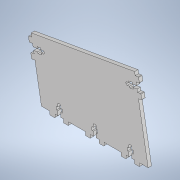
# Autodesk Inventor part: tc_support_down
Saved by Autodesk Inventor 2020 (Build 240168000, 168)
## iProperties
Created: 2019-07-16
Part Number: tc_support_down
Material: Générique
Document SubType Name: Modeling
Designer: Thibault
Density: 1 g/cm^3
Appearance: Par défaut
Author: Thibault
Autodesk Inventor part; units mm, degrees
ref_plane "YZ Plane" through (0, 0, 0) normal (1, 0, 0) x (0, 1, 0)
ref_plane "XZ Plane" through (0, 0, 0) normal (0, 1, 0) x (-1, 0, 0)
ref_plane "XY Plane" through (0, 0, 0) normal (0, 0, 1) x (1, 0, 0)
sketch "Anchor (screw side)" plane through (0, 0, 0) normal (0, 0, 1) x (1, 0, 0)
  circle A0 centre (93.7814, 50.2592) radius 0.85
  line L0 (91.2814, 51.2592) -> (88.2814, 51.2592)
  line L1 (88.2814, 51.2592) -> (88.2814, 49.2592)
  line L2 (88.2814, 49.2592) -> (91.2814, 49.2592)
  line L3 (91.2814, 49.2592) -> (91.2814, 51.2592)
  line L4 (99.2814, 51.2592) -> (96.2814, 51.2592)
  line L5 (96.2814, 51.2592) -> (96.2814, 49.2592)
  line L6 (96.2814, 49.2592) -> (99.2814, 49.2592)
  line L7 (99.2814, 49.2592) -> (99.2814, 51.2592)
  line L8 (91.2814, 51.2592) -> (96.2814, 49.2592) construction
  line L9 (96.2814, 51.2592) -> (91.2814, 49.2592) construction
  line L10 (86.6814, 52.8592) -> (100.8814, 52.8592) construction
  line L11 (100.8814, 52.8592) -> (100.8814, 47.6592) construction
  line L12 (100.8814, 47.6592) -> (86.6814, 47.6592) construction
  line L13 (86.6814, 47.6592) -> (86.6814, 52.8592) construction
  point P0 (103.5798, 50.1132)
  dimension "d27" = 1.7
  dimension "d28" = 3
  dimension "d29" = 2
  dimension "d30" = 3
  dimension "d32" = 5
  dimension "d34" = 1.6
  dimension "d35" = 1.6
  dimension "d36" = 1.6
  dimension "d37" = 1.6
  measures "d27" diameter of A0
  measures "d28" distance of L2.end L1.end
  measures "d29" distance of L1.end L0.end
  measures "d30" distance of L6.end L5.end
  measures "d32" distance between parallel lines of L5 L3
  measures "d34" distance between parallel lines of L0 L10
  measures "d35" distance between parallel lines of L12 L2
  measures "d36" distance between parallel lines of L11 L7
  measures "d37" distance between parallel lines of L13 L1
sketch "Anchor (nut side)" plane through (0, 0, 0) normal (0, 0, 1) x (1, 0, 0)
  line L0 (10, 0) -> (8.35, 0)
  line L1 (8.35, 0) -> (8.35, -2.5)
  line L2 (8.35, -2.5) -> (9.15, -2.5)
  line L3 (9.15, -2.5) -> (9.15, -4.5)
  line L4 (5.85, -4.5) -> (5.85, -2.5)
  line L5 (5.85, -2.5) -> (6.65, -2.5)
  line L6 (6.65, -2.5) -> (6.65, 0)
  line L7 (6.65, 0) -> (5, 0)
  line L8 (2, 0) -> (2, 1.75)
  line L9 (2, 0) -> (3, 0) construction
  line L10 (2.25, 2) -> (4.75, 2)
  line L11 (5, 1.75) -> (5, 0)
  line L12 (5, 2) -> (7, 2) construction
  line L13 (10, 0) -> (10, 1.75)
  line L14 (10.25, 2) -> (12.75, 2)
  line L15 (13, 1.75) -> (13, 0)
  line L16 (0, 0) -> (2, 0)
  line L17 (13, 0) -> (15, 0)
  line L18 (5.85, -4.5) -> (6.65, -4.5)
  line L19 (9.15, -4.5) -> (8.35, -4.5)
  line L20 (6.65, -4.5) -> (6.65, -6)
  line L21 (8.35, -4.5) -> (8.35, -6)
  arc A0 (2.25, 2) -> (2, 1.75) centre (2.25, 1.75) ccw
  arc A1 (5, 1.75) -> (4.75, 2) centre (4.75, 1.75) ccw
  arc A2 (10.25, 2) -> (10, 1.75) centre (10.25, 1.75) ccw
  arc A3 (13, 1.75) -> (12.75, 2) centre (12.75, 1.75) ccw
  line L22 (7.15, -6.5) -> (7.85, -6.5)
  arc A4 (6.65, -6) -> (7.15, -6.5) centre (7.15, -6) ccw
  arc A5 (7.85, -6.5) -> (8.35, -6) centre (7.85, -6) ccw
  point P0 (9.1321, -0.6227)
  point P1 (2, 2)
  point P2 (10, 2)
  point P3 (13, 2)
  point P4 (6.65, -6.5)
  point P5 (8.35, -6.5)
  dimension "d3" = 2
  dimension "d5" = 3
  dimension "d7" = 5
  dimension "d8" = 3
  dimension "d10" = 1.65
  dimension "d11" = 2.5
  dimension "d12" = 0.8
  dimension "d13" = 2
  dimension "d14" = 0.8
  dimension "d15" = 1.7
  dimension "d16" = 2.5
  dimension "d18" = 2
  dimension "d19" = 0.8
  dimension "d20" = 0.8
  dimension "d21" = 2
  dimension "d22" = 2
  dimension "d23" = 1.7
  dimension "d24" = 2
  dimension "d25" = 0.25
  dimension "d38" = 2
  dimension "d39" = 0.5
  measures "d3" distance of point (0, 0) L8.start
  measures "d5" distance of point (2, 2) L12.start
  measures "d7" distance of L7.end L0.start
  measures "d8" distance of point (10, 2) point (13, 2)
  measures "d10" distance of L0.start L0.end
  measures "d11" distance of L0.end L1.end
  measures "d12" distance of L1.end L2.end
  measures "d13" distance of L2.end L3.end
  measures "d14" distance of L4.end L5.end
  measures "d15" distance of L6.end L0.end
  measures "d16" distance of L5.end L6.end
  measures "d18" distance of L15.end point (15, 0)
  measures "d19" distance of L4.start L18.end
  measures "d20" distance of L3.end L19.end
  measures "d21" distance of L18.end point (6.65, -6.5)
  measures "d22" distance of L19.end point (8.35, -6.5)
  measures "d23" distance of L18.end L19.end
  measures "d24" distance of L4.start L4.end
  measures "d25" radius of A0
  measures "d38" distance of the line from the sketch origin of L10
  measures "d39" radius of A4
derived "shared_parameters.ipt"
sketch "Esquisse2" plane through (0, 0, 0) normal (0, 0, 1) x (1, 0, 0)
  line L0 (-14.577, 4.8239) -> (-8.577, 4.8239)
  line L1 (6.423, 4.8239) -> (12.423, 4.8239)
  line L2 (-29.577, 4.8239) -> (-32.577, 4.8239)
  line L3 (27.423, 4.8239) -> (30.423, 4.8239)
  line L4 (-32.577, 4.8239) -> (-32.577, 9.8239)
  line L5 (-32.577, 24.8239) -> (30.423, 24.8239)
  line L6 (30.423, 9.8239) -> (30.423, 4.8239)
  line L7 (-24.577, 4.8239) -> (-22.927, 4.8239)
  line L8 (-22.927, 4.8239) -> (-22.927, 7.3239)
  line L9 (-22.927, 7.3239) -> (-23.727, 7.3239)
  line L10 (-23.727, 7.3239) -> (-23.727, 9.3239)
  line L11 (-20.427, 9.3239) -> (-20.427, 7.3239)
  line L12 (-20.427, 7.3239) -> (-21.227, 7.3239)
  line L13 (-21.227, 7.3239) -> (-21.227, 4.8239)
  line L14 (-21.227, 4.8239) -> (-19.577, 4.8239)
  line L15 (-16.577, 4.8239) -> (-16.577, 3.0739)
  line L16 (-16.577, 4.8239) -> (-17.577, 4.8239) construction
  line L17 (-16.827, 2.8239) -> (-19.327, 2.8239)
  line L18 (-19.577, 3.0739) -> (-19.577, 4.8239)
  line L19 (-19.577, 2.8239) -> (-21.577, 2.8239) construction
  line L20 (-24.577, 4.8239) -> (-24.577, 3.0739)
  line L21 (-24.827, 2.8239) -> (-27.327, 2.8239)
  line L22 (-27.577, 3.0739) -> (-27.577, 4.8239)
  line L23 (-14.577, 4.8239) -> (-16.577, 4.8239)
  line L24 (-27.577, 4.8239) -> (-29.577, 4.8239)
  line L25 (-20.427, 9.3239) -> (-21.227, 9.3239)
  line L26 (-23.727, 9.3239) -> (-22.927, 9.3239)
  line L27 (-21.227, 9.3239) -> (-21.227, 10.8239)
  line L28 (-22.927, 9.3239) -> (-22.927, 10.8239)
  arc A0 (-16.827, 2.8239) -> (-16.577, 3.0739) centre (-16.827, 3.0739) ccw
  arc A1 (-19.577, 3.0739) -> (-19.327, 2.8239) centre (-19.327, 3.0739) ccw
  arc A2 (-24.827, 2.8239) -> (-24.577, 3.0739) centre (-24.827, 3.0739) ccw
  arc A3 (-27.577, 3.0739) -> (-27.327, 2.8239) centre (-27.327, 3.0739) ccw
  line L29 (-21.727, 11.3239) -> (-22.427, 11.3239)
  arc A4 (-21.227, 10.8239) -> (-21.727, 11.3239) centre (-21.727, 10.8239) ccw
  arc A5 (-22.427, 11.3239) -> (-22.927, 10.8239) centre (-22.427, 10.8239) ccw
  line L30 (-3.577, 4.8239) -> (-1.927, 4.8239)
  line L31 (-1.927, 4.8239) -> (-1.927, 7.3239)
  line L32 (-1.927, 7.3239) -> (-2.727, 7.3239)
  line L33 (-2.727, 7.3239) -> (-2.727, 9.3239)
  line L34 (0.573, 9.3239) -> (0.573, 7.3239)
  line L35 (0.573, 7.3239) -> (-0.227, 7.3239)
  line L36 (-0.227, 7.3239) -> (-0.227, 4.8239)
  line L37 (-0.227, 4.8239) -> (1.423, 4.8239)
  line L38 (4.423, 4.8239) -> (4.423, 3.0739)
  line L39 (4.423, 4.8239) -> (3.423, 4.8239) construction
  line L40 (4.173, 2.8239) -> (1.673, 2.8239)
  line L41 (1.423, 3.0739) -> (1.423, 4.8239)
  line L42 (1.423, 2.8239) -> (-0.577, 2.8239) construction
  line L43 (-3.577, 4.8239) -> (-3.577, 3.0739)
  line L44 (-3.827, 2.8239) -> (-6.327, 2.8239)
  line L45 (-6.577, 3.0739) -> (-6.577, 4.8239)
  line L46 (6.423, 4.8239) -> (4.423, 4.8239)
  line L47 (-6.577, 4.8239) -> (-8.577, 4.8239)
  line L48 (0.573, 9.3239) -> (-0.227, 9.3239)
  line L49 (-2.727, 9.3239) -> (-1.927, 9.3239)
  line L50 (-0.227, 9.3239) -> (-0.227, 10.8239)
  line L51 (-1.927, 9.3239) -> (-1.927, 10.8239)
  arc A6 (4.173, 2.8239) -> (4.423, 3.0739) centre (4.173, 3.0739) ccw
  arc A7 (1.423, 3.0739) -> (1.673, 2.8239) centre (1.673, 3.0739) ccw
  arc A8 (-3.827, 2.8239) -> (-3.577, 3.0739) centre (-3.827, 3.0739) ccw
  arc A9 (-6.577, 3.0739) -> (-6.327, 2.8239) centre (-6.327, 3.0739) ccw
  line L52 (-0.727, 11.3239) -> (-1.427, 11.3239)
  arc A10 (-0.227, 10.8239) -> (-0.727, 11.3239) centre (-0.727, 10.8239) ccw
  arc A11 (-1.427, 11.3239) -> (-1.927, 10.8239) centre (-1.427, 10.8239) ccw
  line L53 (17.423, 4.8239) -> (19.073, 4.8239)
  line L54 (19.073, 4.8239) -> (19.073, 7.3239)
  line L55 (19.073, 7.3239) -> (18.273, 7.3239)
  line L56 (18.273, 7.3239) -> (18.273, 9.3239)
  line L57 (21.573, 9.3239) -> (21.573, 7.3239)
  line L58 (21.573, 7.3239) -> (20.773, 7.3239)
  line L59 (20.773, 7.3239) -> (20.773, 4.8239)
  line L60 (20.773, 4.8239) -> (22.423, 4.8239)
  line L61 (25.423, 4.8239) -> (25.423, 3.0739)
  line L62 (25.423, 4.8239) -> (24.423, 4.8239) construction
  line L63 (25.173, 2.8239) -> (22.673, 2.8239)
  line L64 (22.423, 3.0739) -> (22.423, 4.8239)
  line L65 (22.423, 2.8239) -> (20.423, 2.8239) construction
  line L66 (17.423, 4.8239) -> (17.423, 3.0739)
  line L67 (17.173, 2.8239) -> (14.673, 2.8239)
  line L68 (14.423, 3.0739) -> (14.423, 4.8239)
  line L69 (27.423, 4.8239) -> (25.423, 4.8239)
  line L70 (14.423, 4.8239) -> (12.423, 4.8239)
  line L71 (21.573, 9.3239) -> (20.773, 9.3239)
  line L72 (18.273, 9.3239) -> (19.073, 9.3239)
  line L73 (20.773, 9.3239) -> (20.773, 10.8239)
  line L74 (19.073, 9.3239) -> (19.073, 10.8239)
  arc A12 (25.173, 2.8239) -> (25.423, 3.0739) centre (25.173, 3.0739) ccw
  arc A13 (22.423, 3.0739) -> (22.673, 2.8239) centre (22.673, 3.0739) ccw
  arc A14 (17.173, 2.8239) -> (17.423, 3.0739) centre (17.173, 3.0739) ccw
  arc A15 (14.423, 3.0739) -> (14.673, 2.8239) centre (14.673, 3.0739) ccw
  line L75 (20.273, 11.3239) -> (19.573, 11.3239)
  arc A16 (20.773, 10.8239) -> (20.273, 11.3239) centre (20.273, 10.8239) ccw
  arc A17 (19.573, 11.3239) -> (19.073, 10.8239) centre (19.573, 10.8239) ccw
  line L76 (-32.577, 19.8239) -> (-32.577, 18.1739)
  line L77 (-32.577, 18.1739) -> (-30.077, 18.1739)
  line L78 (-30.077, 18.1739) -> (-30.077, 18.9739)
  line L79 (-30.077, 18.9739) -> (-28.077, 18.9739)
  line L80 (-28.077, 15.6739) -> (-30.077, 15.6739)
  line L81 (-30.077, 15.6739) -> (-30.077, 16.4739)
  line L82 (-30.077, 16.4739) -> (-32.577, 16.4739)
  line L83 (-32.577, 16.4739) -> (-32.577, 14.8239)
  line L84 (-32.577, 11.8239) -> (-34.327, 11.8239)
  line L85 (-32.577, 11.8239) -> (-32.577, 12.8239) construction
  line L86 (-34.577, 12.0739) -> (-34.577, 14.5739)
  line L87 (-34.327, 14.8239) -> (-32.577, 14.8239)
  line L88 (-34.577, 14.8239) -> (-34.577, 16.8239) construction
  line L89 (-32.577, 19.8239) -> (-34.327, 19.8239)
  line L90 (-34.577, 20.0739) -> (-34.577, 22.5739)
  line L91 (-34.327, 22.8239) -> (-32.577, 22.8239)
  line L92 (-32.577, 9.8239) -> (-32.577, 11.8239)
  line L93 (-32.577, 22.8239) -> (-32.577, 24.8239)
  line L94 (-28.077, 15.6739) -> (-28.077, 16.4739)
  line L95 (-28.077, 18.9739) -> (-28.077, 18.1739)
  line L96 (-28.077, 16.4739) -> (-26.577, 16.4739)
  line L97 (-28.077, 18.1739) -> (-26.577, 18.1739)
  arc A18 (-34.577, 12.0739) -> (-34.327, 11.8239) centre (-34.327, 12.0739) ccw
  arc A19 (-34.327, 14.8239) -> (-34.577, 14.5739) centre (-34.327, 14.5739) ccw
  arc A20 (-34.577, 20.0739) -> (-34.327, 19.8239) centre (-34.327, 20.0739) ccw
  arc A21 (-34.327, 22.8239) -> (-34.577, 22.5739) centre (-34.327, 22.5739) ccw
  line L98 (-26.077, 16.9739) -> (-26.077, 17.6739)
  arc A22 (-26.577, 16.4739) -> (-26.077, 16.9739) centre (-26.577, 16.9739) ccw
  arc A23 (-26.077, 17.6739) -> (-26.577, 18.1739) centre (-26.577, 17.6739) ccw
  line L99 (30.423, 14.8239) -> (30.423, 16.4739)
  line L100 (30.423, 16.4739) -> (27.923, 16.4739)
  line L101 (27.923, 16.4739) -> (27.923, 15.6739)
  line L102 (27.923, 15.6739) -> (25.923, 15.6739)
  line L103 (25.923, 18.9739) -> (27.923, 18.9739)
  line L104 (27.923, 18.9739) -> (27.923, 18.1739)
  line L105 (27.923, 18.1739) -> (30.423, 18.1739)
  line L106 (30.423, 18.1739) -> (30.423, 19.8239)
  line L107 (30.423, 22.8239) -> (32.173, 22.8239)
  line L108 (30.423, 22.8239) -> (30.423, 21.8239) construction
  line L109 (32.423, 22.5739) -> (32.423, 20.0739)
  line L110 (32.173, 19.8239) -> (30.423, 19.8239)
  line L111 (32.423, 19.8239) -> (32.423, 17.8239) construction
  line L112 (30.423, 14.8239) -> (32.173, 14.8239)
  line L113 (32.423, 14.5739) -> (32.423, 12.0739)
  line L114 (32.173, 11.8239) -> (30.423, 11.8239)
  line L115 (30.423, 24.8239) -> (30.423, 22.8239)
  line L116 (30.423, 11.8239) -> (30.423, 9.8239)
  line L117 (25.923, 18.9739) -> (25.923, 18.1739)
  line L118 (25.923, 15.6739) -> (25.923, 16.4739)
  line L119 (25.923, 18.1739) -> (24.423, 18.1739)
  line L120 (25.923, 16.4739) -> (24.423, 16.4739)
  arc A24 (32.423, 22.5739) -> (32.173, 22.8239) centre (32.173, 22.5739) ccw
  arc A25 (32.173, 19.8239) -> (32.423, 20.0739) centre (32.173, 20.0739) ccw
  arc A26 (32.423, 14.5739) -> (32.173, 14.8239) centre (32.173, 14.5739) ccw
  arc A27 (32.173, 11.8239) -> (32.423, 12.0739) centre (32.173, 12.0739) ccw
  line L121 (23.923, 17.6739) -> (23.923, 16.9739)
  arc A28 (24.423, 18.1739) -> (23.923, 17.6739) centre (24.423, 17.6739) ccw
  arc A29 (23.923, 16.9739) -> (24.423, 16.4739) centre (24.423, 16.9739) ccw
  point P0 (0, 0)
  point P1 (29.9423, 4.944)
  point P2 (-32.577, 24.8239)
  point P3 (-32.577, 3.8239)
  point P4 (30.423, 3.8239)
  dimension "d1" = 10
  dimension "d2" = 10
  dimension "d4" = 3
  dimension "d6" = 3
  dimension "d26" = 90
  dimension "d40" = 20
  constraints: 14 end point, 5 horizontal, 2 vertical, 10 other
  measures "d4" distance of L2.start L2.end
  measures "d6" distance of L3.end L3.start
  measures "d26" angle of L2 L4
extrude "Extrusion1" add sketch "Esquisse2" along normal blind 2
equation "\"d31\" = sheet_thickness"
equation "\"sheet_thickness\" = 2"
